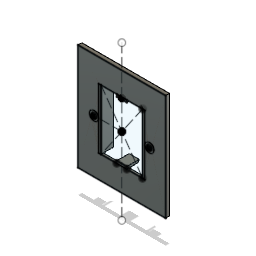
AC Power Connector Module Housing v4 (Autodesk Fusion 360 design; units mm, degrees)
Autodesk Fusion 360 part; units mm, degrees
sketch "Sketch1" plane through (0, 0, 0) normal (0, 0, 1) x (1, 0, 0)
  line L0 (-13.5, 19.5) -> (13.5, 19.5)
  line L1 (13.5, 19.5) -> (13.5, -19.5)
  line L2 (13.5, -19.5) -> (-13.5, -19.5)
  line L3 (-13.5, -19.5) -> (-13.5, 19.5)
  line L4 (-13.5, 19.5) -> (13.5, -19.5) construction
  line L5 (13.5, 19.5) -> (-13.5, -19.5) construction
  line L6 (0, 0) -> (-18, 0) construction
  circle A0 centre (-18, 0) radius 1.4
  circle A1 centre (-18, 0) radius 2.9
  line L7 (0, 50.0244) -> (0, -49.9756) construction
  circle A2 centre (18, 0) radius 2.9
  circle A3 centre (18, 0) radius 1.4
  line L8 (28.5, 34.5) -> (28.5, -34.5)
  line L9 (28.5, -34.5) -> (-28.5, -34.5)
  line L10 (-28.5, -34.5) -> (-28.5, 34.5)
  line L11 (-28.5, 34.5) -> (28.5, 34.5)
  line L12 (-13.5, 19.5) -> (-15, 19.5)
  line L13 (-15, 19.5) -> (-15, -19.5)
  line L14 (-15, -19.5) -> (-13.5, -19.5)
  line L15 (-13.5, -19.5) -> (-13.5, 19.5)
  line L16 (15, -19.5) -> (13.5, -19.5)
  line L17 (15, 19.5) -> (15, -19.5)
  line L18 (13.5, 19.5) -> (15, 19.5)
  line L19 (3.25, 19.5) -> (-3.25, 19.5)
  line L20 (-3.25, 19.5) -> (-3.25, 18)
  line L21 (-3.25, 18) -> (3.25, 18)
  line L22 (3.25, 18) -> (3.25, 19.5)
  line L23 (3.25, 19.5) -> (-3.25, 18) construction
  line L24 (-3.25, 19.5) -> (3.25, 18) construction
  line L25 (-3.25, -19.5) -> (-3.25, -18)
  line L26 (3.25, -18) -> (3.25, -19.5)
  line L27 (-3.25, -18) -> (3.25, -18)
  point P0 (0, 18.75)
  dimension "d2" = 27
  dimension "d3" = 39
  dimension "d4" = -15
  dimension "d5" = 18
  dimension "d6" = 2.8
  dimension "d7" = 1.5
  dimension "d14" = 1.5
  dimension "d19" = 6.5
  dimension "d20" = 1.5
  constraint horizontal L0
  constraint perpendicular L0 L1
  constraint parallel L0 L2
  constraint parallel L1 L3
  constraint coincident L4 L6.start
  constraint coincident L5 L6.start
  constraint coincident L6.start origin
  constraint perpendicular L3 L6
  constraint coincident L6.end A0.centre
  constraint symmetric A0 L7 A3
  constraint symmetric A1 L7 A2
  constraint horizontal L12
  constraint vertical L13
  constraint horizontal L14
  constraint vertical L15
  constraint collinear L2 L14
  constraint symmetric L0.start L7 L0.end
  constraint symmetric L7 L12.end L17.start
  constraint symmetric L7 L13.end L16.start
  constraint symmetric L7 L2.end L1.end
  constraint horizontal L19
  constraint perpendicular L19 L20
  constraint parallel L19 L21
  constraint parallel L20 L22
  constraint coincident L23 P0
  constraint coincident L24 P0
  constraint coincident L7 P0
  constraint collinear L0 L19
  constraint coincident L6.start L7
  constraint vertical L7
  constraint symmetric L6 L19.start L26.end
  constraint symmetric L6 L19.end L25.start
  constraint symmetric L6 L20.end L25.end
  constraint symmetric L6 L21.end L26.start
  measures "d2" distance of L1 L3
  measures "d3" distance of L0.start L2.end
  measures "d5" distance of L6.start L6.end
  measures "d6" diameter of A0
  measures "d14" distance of L13.end L2.end
  measures "d19" distance of L20.end L21.end
  measures "d20" distance of L19.end L20.end
extrude "Extrude1" add sketch "Sketch1" against normal blind 2.5 contours L3 L12 L13 L14 L15 | L1 L16 L17 L18 | A1 | A2 | L8 L9 L10 L11
extrude "Extrude2" add sketch "Sketch1" against normal blind 3 from surface at -2.5 contours A1 | A2
extrude "Extrude3" add sketch "Sketch1" against normal blind 8 contours L3 L12 L13 L14 L15 | L0 L19 L20 L21 L22 | L2 L25 L26 L27 | L1 L16 L17 L18
chamfer "Chamfer2" distance 1 angle 45 2 edges at (15, 0, -8) (-15, 0, -8)
chamfer "Chamfer2" distance 1 angle 45 4 edges at (-8.375, 19.5, -2.5) (8.375, 19.5, -2.5) (8.375, -19.5, -2.5) (-8.375, -19.5, -2.5)
chamfer "Chamfer2" distance 1 angle 45 2 edges at (0, 19.5, -8) (0, -19.5, -8)
equation "d3 = 41 mm - 2 mm"
equation "d5 = ( 36 / 2 ) * 1 mm"
